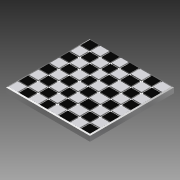
# Autodesk Inventor part: chessboard
Saved by Autodesk Inventor 2015 (Build 190159000, 159)
## iProperties
Created: 2016-04-28
Part Number: chessboard
Material: Generic
Document SubType Name: Modeling
Designer: rosartbrodnitzj3682
Density: 1 g/cm^3
Appearance: Default
Author: rosartbrodnitzj3682
Autodesk Inventor part; units mm, degrees
ref_plane "YZ Plane" through (0, 0, 0) normal (1, 0, 0) x (0, 1, 0)
ref_plane "XZ Plane" through (0, 0, 0) normal (0, 1, 0) x (-1, 0, 0)
ref_plane "XY Plane" through (0, 0, 0) normal (0, 0, 1) x (1, 0, 0)
sketch "Sketch1" plane through (0, 0, 0) normal (0, 1, 0) x (-1, 0, 0)
  line L0 (0, 0) -> (-381, 0)
  line L1 (-381, 0) -> (-381, 381)
  line L2 (-381, 381) -> (0, 381)
  line L3 (0, 381) -> (0, 0)
  dimension "d0" = 381
  dimension "d1" = 381
  constraints: 8 end point, 2 parallel, 1 horizontal, 1 perpendicular
  measures "d0" distance of L2.end L0.start
  measures "d1" distance of L0.start L0.end
extrude "Extrusion1" add sketch "Sketch1" along normal blind 25.4
sketch "Sketch2" plane through (0, 25.4, 0) normal (0, 1, 0) x (1, 0, 0)
  line L0 (381, 0) -> (0, 0) projected
  line L1 (0, 0) -> (0, -381) projected
  line L2 (0, -381) -> (381, -381) projected
  line L3 (381, -381) -> (381, 0) projected
  line L4 (374.65, -6.35) -> (-0.762, -6.35)
  line L5 (-0.762, -6.35) -> (-0.762, -374.65)
  line L6 (-0.762, -374.65) -> (374.65, -374.65)
  line L7 (374.65, -374.65) -> (374.65, -6.35)
  line L8 (6.35, -374.65) -> (6.35, -6.35)
  line L9 (46.736, -6.35) -> (46.736, -374.65)
  line L10 (381, 0) -> (0, 0) projected
  line L11 (93.472, -6.35) -> (93.472, -374.65)
  line L12 (99.822, -374.65) -> (99.822, -6.35)
  line L13 (140.208, -6.35) -> (140.208, -374.65)
  line L14 (180.594, -374.65) -> (180.594, -6.35)
  line L15 (146.558, -6.35) -> (146.558, -374.65)
  line L16 (186.944, -374.65) -> (186.944, -6.35)
  line L17 (281.178, -374.65) -> (281.178, -6.35)
  line L18 (334.264, -374.65) -> (334.264, -6.35)
  line L19 (327.914, -374.65) -> (327.914, -6.35)
  line L20 (287.528, -374.65) -> (287.528, -6.35)
  line L21 (53.086, -374.65) -> (53.086, -6.35)
  line L22 (227.33, -374.65) -> (227.33, -6.35)
  line L23 (233.68, -6.35) -> (233.68, -374.65)
  line L24 (6.35, -334.264) -> (374.65, -334.264)
  line L25 (6.35, -327.914) -> (374.65, -327.914)
  line L26 (374.65, -287.528) -> (6.35, -287.528)
  line L27 (6.35, -281.178) -> (374.65, -281.178)
  line L28 (374.65, -194.056) -> (6.35, -194.056)
  line L29 (6.35, -187.706) -> (374.65, -187.706)
  line L30 (374.65, -100.584) -> (6.35, -100.584)
  line L31 (6.35, -94.234) -> (374.65, -94.234)
  line L32 (374.65, -53.848) -> (6.35, -53.848)
  line L33 (6.35, -47.498) -> (374.65, -47.498)
  line L34 (6.35, -140.97) -> (374.65, -140.97)
  line L35 (374.65, -147.32) -> (6.35, -147.32)
  line L36 (6.35, -240.792) -> (374.65, -240.792)
  line L37 (374.65, -234.442) -> (6.35, -234.442)
  dimension "d5" = 6.35
  dimension "d6" = 6.35
  dimension "d7" = 6.35
  dimension "d8" = 40.386
  dimension "d15" = 6.35
  dimension "d16" = 6.35
  dimension "d20" = 40.386
  dimension "d22" = 40.386
  dimension "d25" = 6.35
  dimension "d26" = 40.386
  dimension "d29" = 6.35
  dimension "d30" = 40.386
  dimension "d31" = 6.35
  dimension "d32" = 6.35
  dimension "d33" = 40.386
  dimension "d34" = 6.35
  dimension "d35" = 6.35
  dimension "d36" = 40.386
  dimension "d39" = 40.386
  dimension "d40" = 6.35
  dimension "d41" = 6.35
  dimension "d42" = 6.35
  dimension "d43" = 6.35
  dimension "d44" = 6.35
  dimension "d45" = 6.35
  dimension "d46" = 6.35
  dimension "d47" = 40.386
  dimension "d48" = 40.386
  dimension "d49" = 40.386
  dimension "d50" = 40.386
  dimension "d51" = 40.386
  dimension "d52" = 40.386
  constraints: 58 end point, 15 vertical, 13 horizontal, 1 parallel, 1 perpendicular, 70 other
  measures "d15" distance between parallel lines of L17 L20
  measures "d16" distance between parallel lines of L18 L19
  measures "d20" distance between parallel lines of L19 L20
  measures "d22" distance between parallel lines of L14 L13
  measures "d29" distance between parallel lines of L11 L12
  measures "d30" distance between parallel lines of L12 L13
  measures "d31" distance between parallel lines of L13 L15
  measures "d32" distance between parallel lines of L9 L21
  measures "d33" distance between parallel lines of L21 L11
  measures "d34" distance between parallel lines of L14 L16
  measures "d35" distance between parallel lines of L23 L22
  measures "d36" distance between parallel lines of L16 L22
  measures "d40" distance between parallel lines of L24 L25
  measures "d41" distance between parallel lines of L27 L26
  measures "d42" distance between parallel lines of L37 L36
  measures "d43" distance between parallel lines of L32 L33
  measures "d44" distance between parallel lines of L30 L31
  measures "d45" distance between parallel lines of L35 L34
  measures "d46" distance between parallel lines of L28 L29
  measures "d47" distance between parallel lines of L26 L25
  measures "d48" distance between parallel lines of L27 L36
  measures "d49" distance between parallel lines of L37 L28
  measures "d50" distance between parallel lines of L29 L35
  measures "d51" distance between parallel lines of L30 L34
  measures "d52" distance between parallel lines of L31 L32
extrude "Extrusion2" cut sketch "Sketch2" against normal blind 5.08 contours L4 L21 L33 L9 | L33 L9 L32 L8 | L9 L24 L21 L6 | L8 L25 L9 L24 | L33 L21 L32 L9 | L9 L25 L21 L24 | L4 L12 L33 L11 | L33 L11 L32 L21 | L32 L21 L31 L9 | L31 L9 L30 L8 | L11 L24 L12 L6 | L21 L25 L11 L24 | L9 L26 L21 L25 | L8 L27 L9 L26 | L33 L12 L32 L11 | L31 L21 L30 L9 | L11 L25 L12 L24 | L9 L27 L21 L26 | L4 L15 L33 L13 | L33 L13 L32 L12 | L32 L12 L31 L11 | L31 L11 L30 L21 | L30 L21 L34 L9 | L34 L9 L35 L8 | L13 L24 L15 L6 | L12 L25 L13 L24 | L11 L26 L12 L25 | L21 L27 L11 L26 | L9 L36 L21 L27 | L8 L37 L9 L36 | L33 L15 L32 L13 | L31 L12 L30 L11 | L34 L21 L35 L9 | L13 L25 L15 L24 | L11 L27 L12 L26 | L9 L37 L21 L36 | L4 L16 L33 L14 | L33 L14 L32 L15 | L32 L15 L31 L13 | L31 L13 L30 L12 | L30 L12 L34 L11 | L34 L11 L35 L21 | L35 L21 L29 L9 | L29 L9 L28 L8 | L14 L24 L16 L6 | L15 L25 L14 L24 | L13 L26 L15 L25 | L12 L27 L13 L26 | L11 L36 L12 L27 | L21 L37 L11 L36 | L9 L28 L21 L37 | L33 L16 L32 L14 | L31 L15 L30 L13 | L34 L12 L35 L11 | L29 L21 L28 L9 | L14 L25 L16 L24 | L13 L27 L15 L26 | L11 L37 L12 L36 | L4 L23 L33 L22 | L33 L22 L32 L16 | L32 L16 L31 L14 | L31 L14 L30 L15 | L30 L15 L34 L13 | L34 L13 L35 L12 | L35 L12 L29 L11 | L29 L11 L28 L21 | L22 L24 L23 L6 | L16 L25 L22 L24 | L14 L26 L16 L25 | L15 L27 L14 L26 | L13 L36 L15 L27 | L12 L37 L13 L36 | L11 L28 L12 L37 | L33 L23 L32 L22 | L31 L16 L30 L14 | L34 L15 L35 L13 | L29 L12 L28 L11 | L22 L25 L23 L24 | L14 L27 L16 L26 | L13 L37 L15 L36 | L4 L20 L33 L17 | L33 L17 L32 L23 | L32 L23 L31 L22 | L31 L22 L30 L16 | L30 L16 L34 L14 | L34 L14 L35 L15 | L35 L15 L29 L13 | L29 L13 L28 L12 | L17 L24 L20 L6 | L23 L25 L17 L24 | L22 L26 L23 L25 | L16 L27 L22 L26 | L14 L36 L16 L27 | L15 L37 L14 L36 | L13 L28 L15 L37 | L33 L20 L32 L17 | L31 L23 L30 L22 | L34 L16 L35 L14 | L29 L15 L28 L13 | L17 L25 L20 L24 | L22 L27 L23 L26 | L14 L37 L16 L36 | L4 L18 L33 L19 | L33 L19 L32 L20 | L32 L20 L31 L17 | L31 L17 L30 L23 | L30 L23 L34 L22 | L34 L22 L35 L16 | L35 L16 L29 L14 | L29 L14 L28 L15 | L19 L24 L18 L6 | L20 L25 L19 L24 | L17 L26 L20 L25 | L23 L27 L17 L26 | L22 L36 L23 L27 | L16 L37 L22 L36 | L14 L28 L16 L37 | L33 L18 L32 L19 | L31 L20 L30 L17 | L34 L23 L35 L22 | L29 L16 L28 L14 | L19 L25 L18 L24 | L17 L27 L20 L26 | L22 L37 L23 L36 | L33 L7 L32 L18 | L32 L18 L31 L19 | L31 L19 L30 L20 | L30 L20 L34 L17 | L34 L17 L35 L23 | L35 L23 L29 L22 | L29 L22 L28 L16 | L18 L25 L7 L24 | L19 L26 L18 L25 | L20 L27 L19 L26 | L17 L36 L20 L27 | L23 L37 L17 L36 | L22 L28 L23 L37 | L31 L18 L30 L19 | L34 L20 L35 L17 | L29 L23 L28 L22 | L19 L27 L18 L26 | L17 L37 L20 L36 | L31 L7 L30 L18 | L30 L18 L34 L19 | L34 L19 L35 L20 | L35 L20 L29 L17 | L29 L17 L28 L23 | L18 L27 L7 L26 | L19 L36 L18 L27 | L20 L37 L19 L36 | L17 L28 L20 L37 | L34 L18 L35 L19 | L29 L20 L28 L17 | L19 L37 L18 L36 | L34 L7 L35 L18 | L35 L18 L29 L19 | L29 L19 L28 L20 | L18 L37 L7 L36 | L19 L28 L18 L37 | L29 L18 L28 L19 | L29 L7 L28 L18
extrude "Extrusion3" cut sketch "Sketch2" against normal blind 0.254 contours L3 L2 L1 L6 L7 L4 L0 | L4 L8 L6 L1
sketch "Sketch3" plane through (381, 0, 381) normal (1, 0, 0) x (0, 0, -1)
  line L0 (374.65, 25.4) -> (374.65, 25.146) projected
  line L1 (374.65, 25.146) -> (381, 22.9643)
  line L2 (381, 22.9643) -> (381, 0)
  line L3 (381, 0) -> (381, 25.146) projected
  line L4 (381, 0) -> (0, 0)
  line L5 (0, 0) -> (381, 0) projected
  line L6 (0, 0) -> (0, 22.9643)
  line L7 (6.35, 25.146) -> (6.35, 20.32) projected
  line L8 (0, 22.9643) -> (6.35, 25.146)
  line L9 (6.35, 25.146) -> (374.65, 25.146)
  line L10 (0, 25.146) -> (381, 25.146) projected
  line L11 (0, 22.9643) -> (0, 25.146)
  line L12 (6.35, 25.146) -> (0, 25.146)
  constraints: 16 end point, 4 collinear, 1 equal length, 1 parallel, 1 perpendicular
extrude "Extrusion4" cut sketch "Sketch3" against normal through all contours L10 L3 L1 | L8 L11 L10
sketch "Sketch4" plane through (381, 0, 0) normal (0, 0, -1) x (-1, 0, 0)
  line L0 (381, 22.9643) -> (0, 22.9643) projected
  line L1 (0, 0) -> (0, 22.9643) projected
  line L2 (381, 0) -> (0, 0) projected
  line L3 (381, 0) -> (381, 22.9643) projected
  line L4 (374.65, 25.4) -> (374.65, 25.146) projected
  line L5 (374.65, 25.146) -> (381, 22.9643)
  line L6 (381, 22.9643) -> (381, 0)
  line L7 (0, 0) -> (381, 0) projected
  line L8 (381, 0) -> (0, 0)
  line L9 (0, 0) -> (0, 22.9643)
  line L10 (6.35, 25.146) -> (0, 22.9643)
  line L11 (6.35, 25.146) -> (374.65, 25.146)
  line L12 (374.65, 25.146) -> (381, 25.146) projected
  line L13 (374.65, 25.146) -> (381, 25.146)
  line L14 (381, 25.146) -> (381, 22.9643)
  line L15 (6.35, 25.146) -> (0, 25.146)
  line L16 (0, 25.146) -> (0, 22.9643)
  constraints: 20 end point, 4 collinear, 3 perpendicular, 1 horizontal
extrude "Extrusion5" cut sketch "Sketch4" against normal through all contours L5 L12 L14 | L16 L15 L10
body "Solid1"
